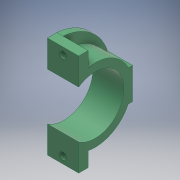
# Autodesk Inventor part: 05-01-Кронштейн верх (update)
Saved by Autodesk Inventor 2018 (Build 220112000, 112)
## iProperties
Part Number: 05-01-Кронштейн верх (update)
Material: Типовые
Document SubType Name: Modeling
Designer: sbnnl
Density: 1 g/cm^3
Appearance: Гладкий — темный цвет морской волны
Author: sbnnl
Autodesk Inventor part; units mm, degrees
ref_plane "YZ Plane" through (0, 0, 0) normal (1, 0, 0) x (0, 1, 0)
ref_plane "XZ Plane" through (0, 0, 0) normal (0, 1, 0) x (-1, 0, 0)
ref_plane "XY Plane" through (0, 0, 0) normal (0, 0, 1) x (1, 0, 0)
sketch "Эскиз1" plane through (0, 0, 0) normal (1, 0, 0) x (0, 1, 0)
  arc A0 (-10.5, -15.2315) -> (-10.5, 15.2315) centre (0, 0) ccw
  line L0 (-18.5, 7.8305) -> (-18.5, -11.8621) construction
  line L1 (-22.5, 35.5109) -> (-22.5, -35.1928) construction
  line L2 (-10.5, 32.5) -> (-10.5, 15.2315)
  line L3 (-4.5, 32.5) -> (-4.5, 23.0651)
  line L4 (-10.5, 32.5) -> (-4.5, 32.5)
  line L5 (-10.5, -32.5) -> (-4.5, -32.5)
  line L6 (0, 0) -> (-8, 0) construction
  arc A1 (-4.5, -23.0651) -> (-4.5, 23.0651) centre (0, 0) ccw
  line L7 (-10.5, -15.2315) -> (-10.5, -32.5)
  line L8 (-4.5, -23.0651) -> (-4.5, -32.5)
  dimension "d0" = 37
  dimension "d2" = 4
  dimension "d3" = 12
  dimension "d4" = 6
  dimension "d5" = 65
  dimension "d6" = 5
  constraints: 18 end point, 6 vertical, 4 perpendicular, 4 point on circle, 2 centre point, 2 coincident, 2 point on line, 1 horizontal, 1 tangent, 1 other
  measures "d0" diameter of A0
  measures "d2" distance between parallel lines of L1 L0
  measures "d3" distance between parallel lines of L2 L1
  measures "d4" distance between parallel lines of L3 L2
  measures "d5" distance between parallel lines of L5 L4
  measures "d6" radial gap between concentric circles of A0 A1
extrude "Выдавливание1" add sketch "Эскиз1" along normal blind 20
sketch "Эскиз2" plane through (0, -4.5, 32.5) normal (0, 1, 0) x (1, 0, 0)
  line L0 (10, -4.2749) -> (10, 72.1744) construction
  line L1 (7.9793, 1) -> (5.9585, 4.5)
  line L2 (5.9585, 4.5) -> (7.9793, 8)
  line L3 (7.9793, 8) -> (12.0207, 8)
  line L4 (12.0207, 8) -> (14.0415, 4.5)
  line L5 (14.0415, 4.5) -> (12.0207, 1)
  line L6 (12.0207, 1) -> (7.9793, 1)
  line L7 (12.0207, 64) -> (14.0415, 60.5)
  line L8 (14.0415, 60.5) -> (12.0207, 57)
  line L9 (12.0207, 57) -> (7.9793, 57)
  line L10 (7.9793, 57) -> (5.9585, 60.5)
  line L11 (5.9585, 60.5) -> (7.9793, 64)
  line L12 (7.9793, 64) -> (12.0207, 64)
  line L13 (0, 32.5) -> (-8.5856, 32.5) construction
  line L14 (0, 65) -> (0, 55.5651) projected
  circle A0 centre (10, 4.5) radius 2.25
  circle A1 centre (10, 60.5) radius 2.25
  point P0 (10, 1)
  point P1 (10, 64)
  dimension "d9" = 7
  dimension "d10" = 56
  dimension "d11" = 10
  dimension "d12" = 4.5
  dimension "d13" = 4.5
  constraints: 28 end point, 4 point on line, 2 centre point, 2 coincident, 2 midpoint, 1 horizontal, 1 parallel, 1 symmetric about line, 1 vertical, 26 other
  measures "d9" distance between parallel lines of L3 L6
  measures "d10" distance of point (10, 60.5) point (10, 4.5)
  measures "d11" distance between parallel lines of L14 L0
  measures "d12" diameter of A0
  measures "d13" diameter of A1
extrude "Выдавливание2" cut sketch "Эскиз2" against normal blind 3
sketch "Эскиз3" plane through (10, -4.5, 28) normal (0, 1, 0) x (1, 0, 0)
  circle A0 centre (0, 0) radius 2.25 projected
  circle A1 centre (0, 56) radius 2.25 projected
  point P0 (-10, 28)
extrude "Выдавливание3" cut sketch "Эскиз3" against normal through all
sketch "Эскиз4" plane through (0, 0, 0) normal (-1, 0, 0) x (0, 0, 1)
  line L0 (-32.5, -10.5) -> (-32.5, -4.5) projected
  line L1 (-32.5, -10.5) -> (-32.5, -9.5)
  line L2 (-32.5, -4.5) -> (-23, -4.5)
  line L3 (32.5, -10.5) -> (15.2315, -10.5) projected
  line L4 (32.5, -10.5) -> (32.5, -4.5)
  line L5 (32.5, -4.5) -> (23, -4.5)
  arc A0 (23.0651, -4.5) -> (-23.0651, -4.5) centre (0, 0) ccw
  arc A1 (32.4076, -10.5) -> (32.5, -9.5) centre (0, -7) ccw
  line L6 (-10.0747, 24) -> (10.0747, 24)
  arc A2 (32.5, -4.5) -> (10.0747, 24) centre (0, -7) ccw
  arc A3 (-10.0747, 24) -> (-32.5, -4.5) centre (0, -7) ccw
  constraints: 11 end point, 9 point on circle, 5 point on line, 4 centre point, 2 horizontal, 1 collinear, 1 perpendicular, 1 vertical
extrude "Выдавливание12" add sketch "Эскиз4" against normal blind 4 contours A3 L6 A2 L5 A0 L2
sketch "Эскиз11" plane through (4, 0, 0) normal (1, 0, 0) x (0, 0, -1)
  line L0 (10.0747, 24) -> (-10.0747, 24) projected
  line L1 (10.0747, 24) -> (-10.0747, 24)
  line L2 (-10.0747, 24) -> (-10.0747, 21)
  arc A0 (32.5, -4.5) -> (10.0747, 24) centre (0, -7) ccw projected
  line L3 (10.0747, 24) -> (10.0747, 21.2309)
  arc A1 (23.0651, -4.5) -> (-23.0651, -4.5) centre (0, 0) ccw projected
  arc A2 (10.0747, 21.2309) -> (-10.0747, 21.2309) centre (0, 0) ccw
  constraints: 6 end point, 3 point on circle, 1 centre point, 1 coincident, 1 collinear, 1 concentric, 1 perpendicular, 1 point on line, 1 vertical
extrude "Выдавливание13" add sketch "Эскиз11" along normal blind 16
sketch "Эскиз12" plane through (0, 24, 10.0747) normal (0, 1, 0) x (1, 0, 0)
  circle A0 centre (15, 10.0747) radius 1
  circle A1 centre (5, 10.0747) radius 1
  point P0 (0, 10.0747)
  dimension "d49" = 2
  constraints: 2 centre point
  measures "d49" diameter of A1
extrude "Выдавливание14" cut sketch "Эскиз12" against normal blind 5
